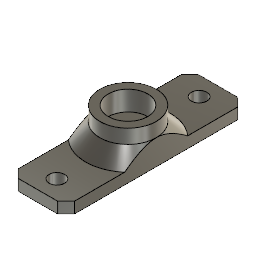
Build Plate Support Bracket (Autodesk Fusion 360 design; units mm, degrees)
description: Build Plate Support Assy
part number: VK-A-BPS
Autodesk Fusion 360 part; units mm, degrees
sketch "Sketch4" plane through (0, 0, 0) normal (0, 0, 1) x (1, 0, 0)
  line L0 (0, 0) -> (20, 0)
  line L1 (20, 0) -> (20, 64)
  line L2 (20, 64) -> (0, 64)
  line L3 (0, 64) -> (0, 0)
  dimension "d47" = 20
  dimension "d48" = 64
  constraint horizontal L0
  constraint vertical L1
  constraint horizontal L2
  constraint vertical L3
  constraint coincident L0.start L3.end
  measures "d47" distance of L0.start L0.end
  measures "d48" distance of L0.start L2.end
extrude "Extrude11" add sketch "Sketch4" along normal blind 4
sketch "Sketch5" plane through (0, 0, 4) normal (0, 0, 1) x (-1, 0, 0)
  line L0 (-20, -64) -> (0, -64)
  line L1 (-20, 0) -> (-20, -64)
  line L2 (0, 0) -> (-20, 0)
  line L3 (0, -64) -> (0, 0)
  line L4 (-10, -64) -> (-10, 0) construction
  circle A0 centre (-10, -32) radius 2.75
  line L5 (-14, -29.6906) -> (-14, -34.3094)
  line L6 (-14, -34.3094) -> (-10, -36.6188)
  line L7 (-10, -36.6188) -> (-6, -34.3094)
  line L8 (-6, -34.3094) -> (-6, -29.6906)
  line L9 (-6, -29.6906) -> (-10, -27.3812)
  line L10 (-10, -27.3812) -> (-14, -29.6906)
  circle A1 centre (-10, -32) radius 7 construction
  circle A2 centre (-10, -32) radius 10
  point P0 (-10, -32)
  dimension "d51" = 5.5
  dimension "d52" = 8
  dimension "d55" = 2.5
  dimension "d718" = 20
  dimension "d719" = 3
  constraint midpoint L0 L4.start
  constraint midpoint L2 L4.end
  constraint midpoint L4 P0
  constraint coincident P0 A0.centre
  constraint vertical L5
  constraint concentric A1 A2
  measures "d51" diameter of A0
  measures "d52" distance of L6 L9
  measures "d718" diameter of A2
  measures "d719" distance of A1 A2
extrude "Extrude12" add sketch "Sketch5" along normal blind 3 contours A2 | L5 L6 L7 L8 L9 L10
extrude "Extrude17" cut sketch "Sketch5" against normal blind 7 contours A0 | L5 L6 L7 L8 L9 L10
sketch "Sketch17" plane through (0, 0, 7) normal (0, 0, 1) x (-1, 0, 0)
  circle A0 centre (-10, -32) radius 2.75
  circle A1 centre (-10, -32) radius 10
  circle A2 centre (-10, -32) radius 7
  dimension "d720" = 3
  constraint concentric A0 A2
  measures "d720" distance of A1 A2
extrude "Extrude31" add sketch "Sketch17" along normal blind 7 contours A1
chamfer "Chamfer7" distance 3 distance2 3 4 edges at (20, 64, 2) (20, 0, 2) (0, 0, 2) (0, 64, 2) measured on face at (20, 32, 1.3333) measured on face at (6.6667, 0, 2.6667) measured on face at (0, 32, 1.3333) measured on face at (13.3333, 64, 2.6667)
sketch "Sketch18" plane through (0, 0, 4) normal (0, 0, 1) x (-1, 0, 0)
  line L0 (-3, -64) -> (0, -61)
  line L1 (0, -61) -> (0, -3)
  line L2 (0, -3) -> (-3, 0)
  line L3 (-17, 0) -> (-20, -3)
  line L4 (-20, -3) -> (-20, -61)
  line L5 (-20, -61) -> (-17, -64)
  circle A0 centre (-10, -32) radius 2.75
  line L6 (-17, -64) -> (-3, -64)
  line L7 (-3, 0) -> (-17, 0)
  line L8 (-10, -57.25) -> (-10, -6.75) construction
  circle A1 centre (-10, -6.75) radius 2.75 construction
  dimension "d726" = 6.75
  dimension "d1087" = 5.5
  dimension "d1088" = 4.25
  constraint parallel L4 L8
  constraint midpoint A0.centre L8
  constraint coincident L8.end A1.centre
  measures "d726" distance of L7 L8.end
  measures "d1087" diameter of A1
hole "Hole1" at (10, 57.25, 4) at (10, 6.75, 4) direction (0, 0, -1) diameter 5.5 depth 17 tip angle 118
chamfer "Chamfer20" distance 5 angle 45 2 edges at (10, 22, 4) (10, 42, 4)
copy_body "Body->Comp2" [suppressed] in component "Bed Support Bracket"
sketch "Sketch1" plane through (0, 0, 14) normal (0, 0, 1) x (-1, 0, 0) in component "Bed Thumb Screw"
  circle A0 centre (-10, -32) radius 2.75
  circle A1 centre (-10, -32) radius 19
  circle A2 centre (-10, -32) radius 6.5
  circle A3 centre (-10, -32) radius 7 construction
  circle A4 centre (-10, -32) radius 13 construction
  point P0 (-10, -32)
  dimension "d741" = 38
  dimension "d747" = 0.5
  dimension "d793" = 0
  dimension "d794" = 0
  dimension "d795" = 0
  dimension "d796" = 0
  dimension "d809" = 0
  dimension "d810" = 0
  dimension "d811" = 0
  dimension "d812" = 0
  dimension "d893" = 0
  dimension "d894" = 0
  dimension "d895" = 0
  dimension "d896" = 0
  dimension "d978" = 13.5
  dimension "d980" = 14
  dimension "d992" = 0
  dimension "d993" = 0
  dimension "d994" = 0
  dimension "d995" = 0
  dimension "d1016" = 26
  dimension "d1053" = 0
  dimension "d1054" = 0
  dimension "d1055" = 0
  dimension "d1056" = 0
  dimension "d1065" = 0
  dimension "d1066" = 0
  dimension "d1067" = 0
  dimension "d1068" = 0
  constraint coincident P0 A0.centre
  constraint concentric A0 A4
  constraint concentric A1 A4
  measures "d741" diameter of A1
  measures "d747" distance of A2 A3
  measures "d980" diameter of A3
  measures "d1016" diameter of A4
extrude "Extrude1" [suppressed] in component "Bed Thumb Screw"
sketch "Sketch2" plane through (0, 0, 7) normal (0, 0, -1) x (1, 0, 0) in component "Bed Thumb Screw"
  circle A0 centre (10, -32) radius 2.75 construction
  circle A1 centre (10, -32) radius 6.5
  line L0 (14, -34.3094) -> (14, -29.6906)
  line L1 (14, -29.6906) -> (10, -27.3812)
  line L2 (10, -27.3812) -> (6, -29.6906)
  line L3 (6, -29.6906) -> (6, -34.3094)
  line L4 (6, -34.3094) -> (10, -36.6188)
  line L5 (10, -36.6188) -> (14, -34.3094)
  point P0 (10, -32)
  dimension "d781" = 8
  constraint coincident P0 A0.centre
  constraint vertical L0
  measures "d781" distance of L1 L4
extrude "Extrude9" [suppressed] in component "Bed Thumb Screw"
extrude "Extrude2" [suppressed] in component "Bed Thumb Screw"
sketch "Sketch7" plane through (0, 0, 14) normal (0, 0, -1) x (1, 0, 0) in component "Bed Thumb Screw"
  circle A0 centre (10, -32) radius 19
  circle A1 centre (10, -32) radius 12
  dimension "d1360" = 24
  constraint concentric A0 A1
  measures "d1360" diameter of A1
extrude "Extrude12'" [suppressed] in component "Bed Thumb Screw"
chamfer "Chamfer1" [suppressed] in component "Bed Thumb Screw"
sketch "Sketch8" plane through (0, 0, 7) normal (0, 0, -1) x (1, 0, 0) in component "Bed Thumb Screw"
  circle A0 centre (10, -32) radius 19
  circle A1 centre (10, -32) radius 12
  circle A2 centre (10, -32) radius 19
  line L0 (10, -32) -> (10, -13) construction
  line L1 (7.5, -13.1652) -> (10, -16)
  line L2 (12.5, -13.1652) -> (10, -16)
  point P0 (10, -32)
  dimension "d1348" = 38
  dimension "d1352" = 3
  dimension "d1353" = 5
  constraint coincident P0 A0.centre
  constraint coincident A0 L0.end
  constraint vertical L0
  constraint coincident A2 L1.start
  constraint coincident L0 L1.end
  constraint coincident A0 L2.start
  constraint symmetric L0 L1.start L2.start
  measures "d1348" diameter of A0
  measures "d1352" distance of L0.end L1.end
  measures "d1353" distance of L1.start L2.start
extrude "Extrude13" [suppressed] in component "Bed Thumb Screw"
fillet "Fillet2" [suppressed] in component "Bed Thumb Screw"
pattern_circular "C-Pattern2" [suppressed] in component "Bed Thumb Screw"
extrude "Extrude10" [suppressed] in component "Bed Thumb Screw"
chamfer "Chamfer4" [suppressed] in component "Bed Thumb Screw"
chamfer "Chamfer5" [suppressed] in component "Bed Thumb Screw"
sketch "Sketch1 (2)" plane through (0, 0, 28) normal (0, 0, 1) x (-1, 0, 0) in component "Bed Corner Support"
  line L0 (5, -47) -> (-25, -47)
  line L1 (-25, -47) -> (-25, -17)
  line L2 (-25, -17) -> (5, -17)
  line L3 (5, -17) -> (5, -47)
  line L4 (-25, -17) -> (5, -47) construction
  line L5 (5, -47) -> (11, -47)
  line L6 (11, -47) -> (11, -11)
  line L7 (11, -11) -> (-25, -11)
  line L8 (-25, -11) -> (-25, -17)
  circle A0 centre (-10, -32) radius 2.75
  circle A1 centre (-10, -32) radius 7.5 construction
  circle A2 centre (-10, -32) radius 8
  dimension "d750" = 30
  dimension "d751" = 30
  dimension "d758" = 6
  dimension "d759" = 6
  dimension "d805" = 0
  dimension "d806" = 0
  dimension "d807" = 0
  dimension "d808" = 0
  dimension "d905" = 0
  dimension "d906" = 0
  dimension "d907" = 0
  dimension "d908" = 0
  dimension "d917" = 0
  dimension "d918" = 0
  dimension "d919" = 0
  dimension "d920" = 0
  dimension "d988" = 0
  dimension "d989" = 0
  dimension "d990" = 0
  dimension "d991" = 0
  dimension "d1049" = 0
  dimension "d1050" = 0
  dimension "d1051" = 0
  dimension "d1052" = 0
  dimension "d1061" = 0
  dimension "d1062" = 0
  dimension "d1063" = 0
  dimension "d1064" = 0
  dimension "d1243" = 0
  dimension "d1244" = 0
  dimension "d1245" = 0
  dimension "d1246" = 0
  dimension "d1299" = 0
  dimension "d1300" = 0
  dimension "d1301" = 0
  dimension "d1302" = 0
  dimension "d1319" = 0
  dimension "d1320" = 0
  dimension "d1321" = 0
  dimension "d1322" = 0
  constraint horizontal L0
  constraint vertical L1
  constraint horizontal L2
  constraint vertical L3
  constraint perpendicular L3 L5
  constraint perpendicular L5 L6
  constraint perpendicular L1 L7
  constraint perpendicular L2 L8
  constraint midpoint L4 A0.centre
  measures "d750" distance of L0.start L0.end
  measures "d751" distance of L0.start L2.end
  measures "d758" distance of L1.end L7.end
  measures "d759" distance of L0.start L5.end
extrude "Extrude1'" [suppressed] in component "Bed Corner Support"
chamfer "Chamfer3" [suppressed] in component "Bed Corner Support"
move_face "OffsetFaces1" [suppressed] in component "Bed Corner Support"
extrude "Extrude2'" [suppressed] in component "Bed Corner Support"
sketch "Sketch19" plane through (0, 17, 0) normal (0, 1, 0) x (-1, 0, 0)
  line L0 (-25, 36) -> (5, 36)
  line L1 (5, 36) -> (5, 46)
  line L2 (5, 46) -> (-25, 46)
  line L3 (-25, 46) -> (-25, 36)
  line L4 (5, 46) -> (-25, 36) construction
  line L5 (-6.8246, 41) -> (-8.4123, 43.75)
  line L6 (-8.4123, 43.75) -> (-11.5877, 43.75)
  line L7 (-11.5877, 43.75) -> (-13.1754, 41)
  line L8 (-13.1754, 41) -> (-11.5877, 38.25)
  line L9 (-11.5877, 38.25) -> (-8.4123, 38.25)
  line L10 (-8.4123, 38.25) -> (-6.8246, 41)
  point P0 (-10, 41)
  dimension "d1092" = 5.5
  constraint coincident L1.end L2.start
  constraint coincident L0.start L3.end
  constraint midpoint L4 P0
  constraint horizontal L9
  measures "d1092" distance of L6 L9
extrude "Extrude4" [suppressed] in component "Bed Corner Support"
sketch "Sketch20" plane through (-5, 0, 0) normal (1, 0, 0) x (0, 1, 0)
  line L0 (17, 36) -> (47, 36)
  line L1 (47, 36) -> (47, 46)
  line L2 (47, 46) -> (17, 46)
  line L3 (17, 46) -> (17, 36)
  line L4 (17, 46) -> (47, 36) construction
  line L5 (33.5877, 38.25) -> (35.1754, 41)
  line L6 (35.1754, 41) -> (33.5877, 43.75)
  line L7 (33.5877, 43.75) -> (30.4123, 43.75)
  line L8 (30.4123, 43.75) -> (28.8246, 41)
  line L9 (28.8246, 41) -> (30.4123, 38.25)
  line L10 (30.4123, 38.25) -> (33.5877, 38.25)
  point P0 (32, 41)
  dimension "d1095" = 5.5
  constraint coincident L2.end L3.start
  constraint coincident L0.end L1.start
  constraint midpoint L4 P0
  constraint horizontal L10
  measures "d1095" distance of L7 L10
extrude "Extrude5" [suppressed] in component "Bed Corner Support"
hole "Hole5" [suppressed] in component "Bed Corner Support"
hole "Hole6" [suppressed] in component "Bed Corner Support"
chamfer "Chamfer2" [suppressed] in component "Bed Corner Support"
chamfer "Chamfer4'" [suppressed] in component "Bed Corner Support"
chamfer "Chamfer1'" [suppressed] in component "Bed Corner Support"
equation "d751 = d750"
equation "d759 = d758"
named bodies: "Bottom Bed Support", "Bed Support Bracket", "Bed Thumb Screw", "Bed Corner Support"
